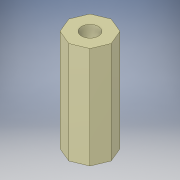
# Autodesk Inventor part: separator
Saved by Autodesk Inventor 2019 (Build 230136000, 136)
## iProperties
Created: 2019-04-09
Part Number: separator
Material: PET Plastic
Document SubType Name: Modeling
Designer: jmc
Density: 1.541 g/cm^3
Appearance: Smooth - Ash
Author: jmc
## iProperties of the stored document separator_3DPrint.ipt
Created: 2019-04-09
Part Number: separator_3DPrint
Material: Generic
Document SubType Name: Modeling
Designer: jmc
Density: 1 g/cm^3
Appearance: Default
Author: jmc
Autodesk Inventor part; units mm, degrees
ref_plane "YZ Plane" through (0, 0, 0) normal (1, 0, 0) x (0, 1, 0)
ref_plane "XZ Plane" through (0, 0, 0) normal (0, 1, 0) x (-1, 0, 0)
ref_plane "XY Plane" through (0, 0, 0) normal (0, 0, 1) x (1, 0, 0)
sketch "Sketch1" plane through (0, 0, 0) normal (0, 1, 0) x (-1, 0, 0)
  circle A0 centre (0, 0) radius 2.5 construction
  line L0 (-2.5, 0) -> (-1.7678, 1.7678)
  line L1 (-1.7678, 1.7678) -> (0, 2.5)
  line L2 (0, 2.5) -> (1.7678, 1.7678)
  line L3 (1.7678, 1.7678) -> (2.5, 0)
  line L4 (2.5, 0) -> (1.7678, -1.7678)
  line L5 (1.7678, -1.7678) -> (0, -2.5)
  line L6 (0, -2.5) -> (-1.7678, -1.7678)
  line L7 (-1.7678, -1.7678) -> (-2.5, 0)
  point P0 (0, -2.5)
  dimension "d0" = 5
  constraints: 16 end point, 3 coincident, 2 point on circle, 1 centre point, 17 other
  measures "d0" diameter of A0
extrude "Extrusion1" add sketch "Sketch1" along normal blind 12
sketch "Sketch4" plane through (0, 12, 0) normal (0, 1, 0) x (1, 0, 0)
  line L0 (1.7678, -1.7678) -> (2.5, 0) construction
  line L1 (2.5, 0) -> (1.7678, 1.7678) construction
  line L2 (1.7678, 1.7678) -> (0, 2.5) construction
  line L3 (0, 2.5) -> (-1.7678, 1.7678) construction
  line L4 (-1.7678, 1.7678) -> (-2.5, 0) construction
  line L5 (-2.5, 0) -> (-1.7678, -1.7678) construction
  line L6 (-1.7678, -1.7678) -> (0, -2.5) construction
  line L7 (0, -2.5) -> (1.7678, -1.7678) construction
  circle A0 centre (0, 0) radius 2.5 construction
  constraints: 1 coincident, 1 horizontal alignment, 2 other
hole "Hole2" at (0, 12, 0) direction (0, -1, 0) diameter 2 depth 7
body "Solid1"
